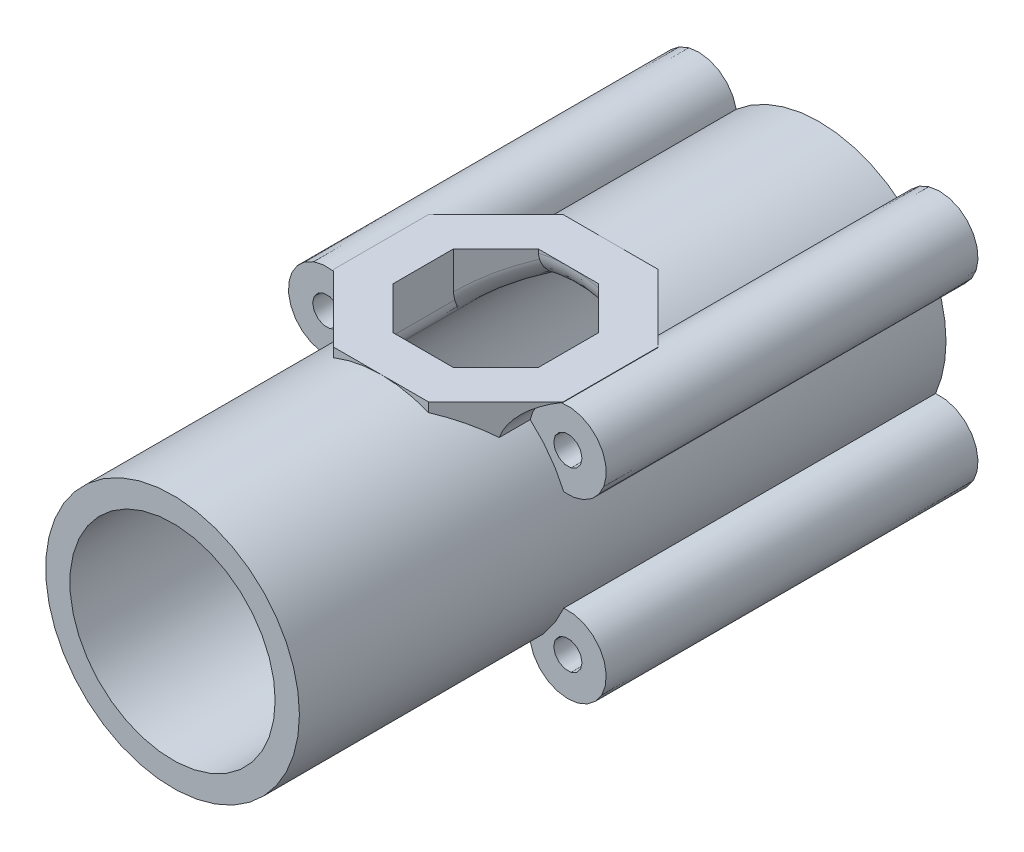
# Autodesk Inventor part: Dispensador V3.2
Saved by Autodesk Inventor 2020.3 (Build 243373000, 373)
## iProperties
Created: 2021-01-23
Part Number: Dispensador V3.2
Material: Generic
Document SubType Name: Modeling
Designer: juanp
Density: 1 g/cm^3
Appearance: Default
Author: juanp
Autodesk Inventor part; units mm, degrees
ref_plane "YZ Plane" through (0, 0, 0) normal (1, 0, 0) x (0, 1, 0)
ref_plane "XY Plane" through (0, 0, 0) normal (0, 0, 1) x (1, 0, 0)
sketch "Sketch1" plane through (0, 0, 0) normal (0, 0, 1) x (1, 0, 0)
  circle A0 centre (0, 0) radius 12.7
  circle A1 centre (0, 0) radius 15.7
  dimension "d4" = 25.4
  dimension "d13" = 3
  constraints: 2 centre point, 2 coincident
  measures "d4" diameter of A0
  measures "d13" radial gap between concentric circles of A1 A0
extrude "Extrusion1" add sketch "Sketch1" along normal mid plane 80
sketch "Sketch2" plane through (0, 0, 0) normal (0, 1, 0) x (-1, 0, 0)
  line L0 (-3.719744, 8.980256) -> (3.719744, 8.980256)
  line L1 (3.719744, 8.980256) -> (8.980256, 3.719744)
  line L2 (8.980256, 3.719744) -> (8.980256, -3.719744)
  line L3 (8.980256, -3.719744) -> (3.719744, -8.980256)
  line L4 (3.719744, -8.980256) -> (-3.719744, -8.980256)
  line L5 (-3.719744, -8.980256) -> (-8.980256, -3.719744)
  line L6 (-8.980256, -3.719744) -> (-8.980256, 3.719744)
  line L7 (-8.980256, 3.719744) -> (-3.719744, 8.980256)
  line L8 (12.7, 40) -> (12.7, -40) construction
  line L9 (-12.7, 40) -> (-12.7, -40) construction
  point P0 (0, 0)
  point P1 (0, 0)
  dimension "d28" = 3.71974
  constraints: 16 end point, 1 coincident, 1 vertical, 17 other
  measures "d28" distance between parallel lines of L6 L9
extrude "Extrusion2" cut sketch "Sketch2" along normal through all
fillet "Fillet2" radius 3 10 edges at (-6.544, 10.8842, 6.156) (-8.9803, 8.9803, -1.8599) (-8.9803, 8.9803, 1.8599) (-6.544, 10.8842, -6.156) (0, 12.7, 8.9803) (0, 12.7, -8.9803) (6.544, 10.8842, 6.156) (8.9803, 8.9803, 1.8599) (8.9803, 8.9803, -1.8599) (6.544, 10.8842, -6.156)
sketch "Sketch3" plane through (0, 0, 0) normal (0, 0, 1) x (1, 0, 0)
  circle A0 centre (0, 0) radius 15.7
  line L0 (14.911321, 15.7) -> (-14.911321, 15.7) construction
  arc A1 (14.412626, 6.226251) -> (10.254882, 11.88812) centre (14.911321, 10.95) ccw
  arc A2 (10.254882, -11.88812) -> (14.412626, -6.226251) centre (14.911321, -10.95) ccw
  circle A3 centre (14.911321, 10.95) radius 1.75
  circle A4 centre (14.911321, -10.95) radius 1.75
  circle A5 centre (14.911321, -10.95) radius 2.8 construction
  circle A6 centre (14.911321, 10.95) radius 2.8 construction
  line L1 (0, 0) -> (14.911321, 10.95) construction
  line L2 (14.911321, 10.95) -> (14.911321, 0) construction
  line L3 (14.911321, 0) -> (14.911321, -10.95) construction
  line L4 (14.911321, -10.95) -> (0, 0) construction
  line L5 (0, 0) -> (14.911321, 0) construction
  line L6 (0, 0) -> (0, 15.7) construction
  line L7 (0, 0) -> (-14.911321, 0) construction
  line L8 (0, 0) -> (-14.911321, 10.95) construction
  line L9 (-14.911321, 10.95) -> (-14.911321, 0) construction
  line L10 (-14.911321, 0) -> (-14.911321, -10.95) construction
  line L11 (-14.911321, -10.95) -> (0, 0) construction
  circle A7 centre (-14.911321, 10.95) radius 2.8 construction
  circle A8 centre (-14.911321, -10.95) radius 2.8 construction
  circle A9 centre (-14.911321, -10.95) radius 1.75
  circle A10 centre (-14.911321, 10.95) radius 1.75
  arc A11 (-10.254882, 11.88812) -> (-14.412626, 6.226251) centre (-14.911321, 10.95) ccw
  arc A12 (-14.412626, -6.226251) -> (-10.254882, -11.88812) centre (-14.911321, -10.95) ccw
  dimension "d54" = 5.6
  dimension "d56" = 3.5
  dimension "d57" = 3
  constraints: 24 end point, 12 centre point, 12 coincident, 10 point on circle, 9 equal radius, 4 equal length, 4 horizontal, 2 point on line, 2 vertical, 1 midpoint, 1 tangent, 12 other
  measures "d54" diameter of A6
  measures "d56" diameter of A3
  measures "d57" radial gap between concentric circles of A1 A3
extrude "Extrusion3" add sketch "Sketch3" along normal blind 6 and the other way blind 40 contours A0 A1 | A2 A0 | A0 A11 | A12 A0
ref_plane "Work Plane1" through (0, 15.7, 0) normal (0, 1, 0) x (-1, 0, 0)
sketch "Sketch4" plane through (0, 15.7, 0) normal (0, 1, 0) x (-1, 0, 0)
  line L0 (14.2, -5.881833) -> (5.881833, -14.2)
  line L1 (5.881833, -14.2) -> (-5.881833, -14.2)
  line L2 (-5.881833, -14.2) -> (-14.2, -5.881833)
  line L3 (-14.2, -5.881833) -> (-14.2, 5.881833)
  line L4 (-14.2, 5.881833) -> (-5.881833, 14.2)
  line L5 (-5.881833, 14.2) -> (5.881833, 14.2)
  line L6 (5.881833, 14.2) -> (14.2, 5.881833)
  line L7 (14.2, 5.881833) -> (14.2, -5.881833)
  line L8 (10.254882, -9.826951) -> (10.254882, 9.826951)
  line L9 (-10.254882, -9.826951) -> (-10.254882, 9.826951)
  line L10 (10.254882, -40) -> (10.254882, 6) construction
  line L11 (-10.254882, 6) -> (-10.254882, -40) construction
  line L12 (8.980256, 3.719744) -> (8.980256, -3.719744)
  line L13 (8.980256, -3.719744) -> (3.719744, -8.980256)
  line L14 (3.719744, -8.980256) -> (-3.719744, -8.980256)
  line L15 (-3.719744, -8.980256) -> (-8.980256, -3.719744)
  line L16 (-8.980256, -3.719744) -> (-8.980256, 3.719744)
  line L17 (-8.980256, 3.719744) -> (-3.719744, 8.980256)
  line L18 (-3.719744, 8.980256) -> (3.719744, 8.980256)
  line L19 (3.719744, 8.980256) -> (8.980256, 3.719744)
  line L20 (-3.719744, -8.980256) -> (3.719744, -8.980256)
  point P0 (0, 0)
  point P1 (0, 0)
  point P2 (0, 0)
  dimension "d62" = 28.4
  constraints: 36 end point, 4 point on line, 3 collinear, 2 coincident, 2 vertical, 1 parallel, 34 other
  measures "d62" distance between parallel lines of L7 L3
extrude "Extrusion4" add sketch "Sketch4" against normal up to surface contours L0 L1 L2 L9 L4 L5 L6 L8 round surface about axis through (0, 0, 0) along (0, 0, 1) radius 15.7 far side no
extrude "Extrusion5" add sketch "Sketch4" against normal up to surface contours L2 L3 L4 L9 round surface about axis through (14.911321, 10.95, 0) along (0, 0, 1) radius 4.75 far side no
extrude "Extrusion6" add sketch "Sketch4" against normal up to surface contours L0 L8 L6 L7 round surface about axis through (-14.911321, 10.95, 0) along (0, 0, 1) radius 4.75 far side no
equation "\"d4\" = diametro_interno"
equation "\"d13\" = grosor_pared"
equation "\"d15\" = longitud_efectiva"
equation "\"d28\" = 0.146447 * diametro_interno"
equation "\"d53\" = grosor_pared"
equation "\"d54\" = m3_tuerca_largo + tolerancia_inserto"
equation "\"d56\" = m3_diametro + tolerancia_agujero"
equation "\"d57\" = grosor_pared"
equation "\"d58\" = grosor_pared + m3_altura_cabeza"
equation "\"d59\" = 0.5 * longitud_efectiva"
equation "\"d62\" = diametro_interno + grosor_pared"
equation "\"grosor_pared\" = 3"
equation "\"diametro_interno\" = 25.4"
equation "\"longitud_efectiva\" = 80"
equation "\"tolerancia_agujero\" = 0.5"
equation "\"tolerancia_inserto\" = 0.2"
equation "\"m3_diametro\" = 3"
equation "\"m3_tuerca_largo\" = 5.4"
equation "\"celdacarga_ancho\" = 12.7"
equation "\"celdacarga_separacion_huecos\" = 15"
equation "\"tornillo_diametro_eje\" = 5"
equation "\"d0\" = diametro_interno"
equation "\"d1\" = grosor_pared"
equation "\"d3\" = 0"
equation "\"d5\" = 0"
equation "\"d6\" = m3_diametro + tolerancia_agujero"
equation "\"d7\" = grosor_pared"
equation "\"d8\" = m3_tuerca_largo + tolerancia_inserto"
equation "\"d9\" = 0.207107 * diametro_interno + 0.414214 * grosor_pared"
equation "\"d10\" = 0"
equation "\"d11\" = 0.5 * longitud_efectiva + grosor_pared"
equation "\"d12\" = 0"
equation "\"d14\" = 0"
equation "\"d16\" = 0"
equation "\"d18\" = 0"
equation "\"d20\" = 0"
equation "\"d22\" = 0"
equation "\"i3d_altura_capa\" = 0.3"
equation "\"d23\" = 2 * grosor_pared + celdacarga_separacion_huecos + tolerancia_agujero + m3_diametro"
equation "\"d24\" = m3_diametro + tolerancia_agujero"
equation "\"d25\" = 15"
equation "\"d26\" = celdacarga_ancho"
equation "\"d27\" = 0"
equation "\"d29\" = 0"
equation "\"d30\" = grosor_pared"
equation "\"d31\" = 0"
equation "\"d34\" = 0"
equation "\"d35\" = grosor_pared"
equation "\"d37\" = 0"
equation "\"d38\" = tornillo_diametro_eje + tolerancia_agujero"
equation "\"d39\" = 0.207107 * diametro_interno + 0.414214 * grosor_pared"
equation "\"d40\" = 0.5 * longitud_efectiva + grosor_pared"
equation "\"d41\" = 0"
equation "\"d42\" = 0"
equation "\"m3_diametro_cabeza\" = 5.4"
equation "\"m3_altura_cabeza\" = 3"
equation "\"d44\" = 1000000"
equation "\"d45\" = 0"
equation "\"d46\" = m3_altura_cabeza"
equation "\"d47\" = 0"
equation "\"d48\" = -grosor_pared"
equation "\"m3_tuerca_alto\" = 2.5"
equation "\"d74\" = 6.503"
equation "\"d93\" = grosor_pared"
equation "\"d96\" = tolerancia_agujero + m3_diametro + 2 * grosor_pared"
equation "\"d97\" = 0.5 * diametro_interno + grosor_pared"
equation "\"d98\" = grosor_pared"
equation "\"d99\" = 0"
equation "\"d100\" = 4 * tolerancia_agujero"
equation "\"d101\" = tolerancia_agujero + m3_diametro + 2 * grosor_pared"
equation "\"d103\" = 0"
equation "\"d104\" = 4 * tolerancia_agujero"
equation "\"d106\" = 0"
equation "\"mg996r_distancia_par_huecos\" = 49.422"
equation "\"mg996r_distancia_eje_huecoslejanos\" = 34.811"
equation "\"mg996r_distancia_huecos\" = 9.85"
equation "\"mg996r_diametro_hueco\" = 1.25"
equation "\"d107\" = m3_tuerca_largo + tolerancia_inserto"
equation "\"d109\" = m3_tuerca_alto"
equation "\"d110\" = 0"
equation "\"d111\" = grosor_pared"
equation "\"d114\" = grosor_pared"
equation "\"d115\" = 0"
equation "\"d121\" = 0"
equation "\"d122\" = 90deg"
equation "\"d123\" = 0"
equation "\"d124\" = 90deg"
equation "\"d125\" = 0"
equation "\"d126\" = 90deg"
equation "\"d127\" = 0"
equation "\"d128\" = 90deg"
equation "\"grosor_embudo\" = 1"
equation "\"d130\" = 0"
equation "\"d131\" = m3_tuerca_largo + tolerancia_inserto"
equation "\"d133\" = m3_tuerca_alto"
equation "\"d134\" = 0"
equation "\"d138\" = 45deg"
equation "\"d139\" = diametro_interno"
equation "\"d141\" = 0"
equation "\"d142\" = 0.5"
equation "\"d143\" = 0.5"
equation "\"d144\" = 0.5 * ancho_salida"
equation "\"d148\" = 0.333333 * grosor_pared"
equation "\"d149\" = 0.333333 * grosor_pared"
equation "\"d150\" = 0"
equation "\"d151\" = 0.333333 * grosor_pared"
equation "\"d154\" = 0"
equation "\"d43\" = m3_diametro_cabeza + tolerancia_inserto"
equation "\"d85\" = mg996r_distancia_eje_huecoslejanos"
equation "\"d86\" = mg996r_distancia_par_huecos"
equation "\"d87\" = mg996r_distancia_huecos"
equation "\"d88\" = mg996r_diametro_hueco"
equation "\"d117\" = grosor_embudo"
equation "\"d119\" = grosor_embudo"
equation "\"d19\" = i3d_altura_puente_grueso"
equation "\"d21\" = i3d_altura_puente_delgado + i3d_altura_puente_grueso"
equation "\"ancho_salida\" = 10"
equation "\"i3d_altura_puente_grueso\" = 0.65"
equation "\"i3d_altura_puente_delgado\" = 0.35"
body "Solid1"
